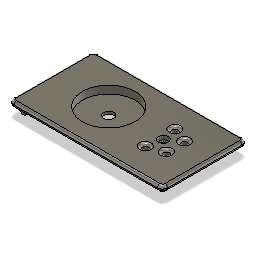
pluggable-12v-dimmer (Autodesk Fusion 360 design; units mm, degrees)
Autodesk Fusion 360 part; units mm, degrees
note: some values were not read from the file. Chosen so that the rebuilt part matches the saved one: which bodies a step acts on. Set by a fixed rule: which face or edge a step refers to.
sketch "pcb" plane through (0, 0, 0) normal (0, 1, 0) x (1, 0, 0) in component "Logic board"
  line L0 (0, 0) -> (53, 0)
  line L1 (53, 0) -> (53, -40)
  line L2 (53, -40) -> (0, -40)
  line L3 (0, -40) -> (0, 0)
  dimension "d1" = 53
  dimension "d2" = 40
  constraint horizontal L0
  constraint vertical L1
  constraint horizontal L2
  constraint vertical L3
  constraint coincident L0.start L3.end
  measures "d1" distance of L0.start L0.end
  measures "d2" distance of L0.start L2.end
sketch "esp32" plane through (0, 0, 0) normal (0, 1, 0) x (-1, 0, 0) in component "Logic board"
  line L0 (-3, -5) -> (-32, -5)
  line L1 (-32, -5) -> (-32, 47)
  line L2 (-32, 47) -> (-3, 47)
  line L3 (-3, 47) -> (-3, -5)
  dimension "d3" = 29
  dimension "d4" = 52
  constraint horizontal L0
  constraint vertical L1
  constraint horizontal L2
  constraint vertical L3
  measures "d3" distance of L0.start L0.end
  measures "d4" distance of L0.start L2.end
sketch "rotary enc" plane through (0, 0, 0) normal (0, 1, 0) x (1, 0, 0) in component "Logic board"
  circle A0 centre (40, -22) radius 6.5
  circle A1 centre (40, -22) radius 3.4
  point P0 (40, -22)
  dimension "d5" = 13
  dimension "d6" = 6.8
  constraint concentric A0 A1
  constraint coincident P0 A0.centre
  measures "d5" diameter of A0
  measures "d6" diameter of A1
sketch "Pololu" plane through (0, 0, 0) normal (0, 1, 0) x (1, 0, 0) in component "Logic board"
  line L0 (33, -15) -> (50, -15)
  line L1 (50, -15) -> (50, -2)
  line L2 (50, -2) -> (33, -2)
  line L3 (33, -2) -> (33, -15)
  dimension "d7" = 17
  constraint horizontal L0
  constraint vertical L1
  constraint horizontal L2
  constraint vertical L3
  measures "d7" distance of L0.start L0.end
sketch "mosfet" plane through (0, 0, 0) normal (0, 1, 0) x (1, 0, 0) in component "Logic board"
  line L0 (40, -30) -> (59, -30)
  line L1 (59, -30) -> (59, -39)
  line L2 (59, -39) -> (40, -39)
  line L3 (40, -39) -> (40, -30)
  constraint horizontal L0
  constraint vertical L1
  constraint horizontal L2
  constraint vertical L3
extrude "Extrude1" add sketch "pcb" against normal blind 2.5 makes body 1 in component "Logic board"
extrude "Extrude2" add sketch "esp32" along normal blind 7.5 bodies 1 in component "Logic board"
extrude "Extrude3" add sketch "rotary enc" sketch "mosfet" sketch "Pololu" along normal blind 6 contours A0 | A1 of sketch 2 of sketch 3 bodies 1 in component "Logic board"
extrude "Extrude4" add sketch "rotary enc" along normal blind 17.5 separate body contours A1 makes body 2 in component "Logic board"
sketch "jumper" plane through (0, 0, 0) normal (0, 1, 0) x (1, 0, 0) in component "Logic board"
  line L0 (50, -16) -> (52, -16)
  line L1 (52, -16) -> (52, -19)
  line L2 (52, -19) -> (50, -19)
  line L3 (50, -19) -> (50, -16)
  constraint horizontal L0
  constraint vertical L1
  constraint horizontal L2
  constraint vertical L3
extrude "Extrude5" add sketch "jumper" along normal blind 10 bodies 1 in component "Logic board"
combine "Combine1" operation add target body 1 tool bodies 2 in component "Logic board"
sketch "Sketch1" plane through (0, 0, 0) normal (0, 1, 0) x (1, 0, 0) in component "PTT stekker"
  line L0 (51.8, -11.4201) -> (51.8, -30.6799)
  line L1 (20.5424, -1.0921) -> (51.8, -11.4201)
  line L2 (20.5424, -41.0079) -> (51.8, -30.6799)
  arc A0 (20.5424, -1.0921) -> (20.5424, -41.0079) centre (21.0782, -21.05) ccw
  circle A1 centre (19.6032, -9.55) radius 2
  circle A2 centre (19.6032, -32.55) radius 2
  circle A3 centre (31.0676, -13.85) radius 2
  circle A4 centre (31.0676, -28.25) radius 2
  line L3 (21.0782, -40.35) -> (15.9681, -40.35)
  line L4 (21.0782, -40.35) -> (22.5334, -40.35)
  line L5 (21.0782, -1.75) -> (15.488, -1.8836)
  line L6 (21.0782, -1.75) -> (22.5334, -1.75)
  circle A5 centre (21.0782, -21.05) radius 4
  circle A6 centre (21.0782, -21.05) radius 2
  point P0 (19.6032, -9.55)
  point P1 (31.0676, -13.85)
  point P2 (31.0676, -28.25)
  point P3 (19.6032, -32.55)
  point P4 (21.0782, -21.05)
  dimension "d24" = 4
  dimension "d25" = 4
  dimension "d26" = 4
  dimension "d27" = 4
  dimension "d28" = 19.3
  dimension "d29" = 19.3
  dimension "d110" = 8
  dimension "d111" = 4
  constraint vertical L0
  constraint coincident P0 A1.centre
  constraint coincident P3 A2.centre
  constraint coincident P1 A3.centre
  constraint coincident P2 A4.centre
  constraint coincident A0 L3.end
  constraint coincident L2 L4.end
  constraint coincident A0 L5.end
  constraint coincident L1 L6.end
  constraint concentric A0 A5
  constraint concentric A0 A6
  constraint coincident P4 A0.centre
  measures "d24" diameter of A1
  measures "d25" diameter of A2
  measures "d26" diameter of A3
  measures "d27" diameter of A4
  measures "d28" distance of P4 L3.start
  measures "d29" distance of P4 L5.start
  measures "d110" diameter of A5
  measures "d111" diameter of A6
extrude "Extrude1'" add sketch "Sketch1" against normal blind 19.5 separate body contours A1 | A2 | A3 | A4 makes body 3 at (33.0651, -13, 28.3497) makes body 4 at (33.0651, -13, 13.9497) makes body 5 at (21.6007, -13, 32.6497) makes body 6 at (21.6007, -13, 9.6497) in component "PTT stekker"
extrude "Extrude2'" add sketch "Sketch1" along normal blind 12.5 contours L0 L1 L2 A0 L3 L4 L5 L6 | L1 A0 L5 L6 | L2 A0 L3 L4 | A1 | A2 | A3 | A4 | A5 | A6 bodies 3 4 5 6 in component "PTT stekker"
extrude "Extrude3'" cut sketch "Sketch1" along normal blind 9 contours L1 A0 L5 L6 | L2 A0 L3 L4 bodies 3 in component "PTT stekker"
extrude "Extrude4'" cut sketch "Sketch1" along normal blind 22 contours A6 bodies 3 in component "PTT stekker"
fillet "Fillet1" radius 2 4 edges at (29.2029, -19.5, 27.5268) (17.7386, -19.5, 31.8268) (17.7386, -19.5, 8.8268) (29.2029, -19.5, 13.1268) on bodies 3 4 5 6 in component "PTT stekker"
sketch "Sketch1 (2)" plane through (0, 0, 0) normal (0, 1, 0) x (1, 0, 0) in component "PTT stopcontact"
  line L0 (4, 0) -> (57.5, 0)
  line L1 (61.5, -4) -> (61.5, -57.5)
  line L2 (57.5, -61.5) -> (4, -61.5)
  line L3 (0, -57.5) -> (0, -4)
  arc A0 (4, 0) -> (0, -4) centre (4, -4) ccw
  arc A1 (61.5, -4) -> (57.5, 0) centre (57.5, -4) ccw
  arc A2 (57.5, -61.5) -> (61.5, -57.5) centre (57.5, -57.5) ccw
  arc A3 (0, -57.5) -> (4, -61.5) centre (4, -57.5) ccw
  circle A4 centre (29, -42.5) radius 3.5
  circle A5 centre (41, -38.4) radius 3.5
  circle A6 centre (41, -23.6) radius 3.5
  circle A7 centre (29, -19.5) radius 3.5
  circle A8 centre (29, -19.5) radius 2.2
  circle A9 centre (41, -23.6) radius 2.2
  circle A10 centre (29, -42.5) radius 2.2
  circle A11 centre (41, -38.4) radius 2.2
  line L4 (32.3924, -18.6389) -> (57.8397, -18.6389) construction
  circle A12 centre (31.4907, -30.8181) radius 3
  circle A13 centre (31.4907, -30.8181) radius 1.25
  arc A14 (59.75, -4) -> (57.5, -1.75) centre (57.5, -4) ccw
  line L5 (4, -1.75) -> (57.5, -1.75)
  arc A15 (4, -1.75) -> (1.75, -4) centre (4, -4) ccw
  line L6 (1.75, -57.5) -> (1.75, -4)
  arc A16 (1.75, -57.5) -> (4, -59.75) centre (4, -57.5) ccw
  line L7 (57.5, -59.75) -> (4, -59.75)
  arc A17 (57.5, -59.75) -> (59.75, -57.5) centre (57.5, -57.5) ccw
  line L8 (59.75, -4) -> (59.75, -57.5)
  line L9 (31.4907, -30.8181) -> (31.4907, -50.8681)
  line L10 (31.4907, -30.8181) -> (31.4907, -10.7681)
  circle A18 centre (31.4907, -50.8681) radius 2
  circle A19 centre (31.4907, -10.7681) radius 2
  point P0 (61.5, 0)
  point P1 (0, -61.5)
  point P2 (29, -19.5)
  point P3 (41, -23.6)
  point P4 (41, -38.4)
  point P5 (29, -42.5)
  dimension "d39" = 61.5
  dimension "d40" = 61.5
  dimension "d41" = 4
  dimension "d42" = 7
  dimension "d43" = 7
  dimension "d44" = 7
  dimension "d45" = 7
  dimension "d46" = 4.4
  dimension "d47" = 4.4
  dimension "d48" = 4.4
  dimension "d49" = 4.4
  dimension "d52" = 6
  dimension "d53" = 2.5
  dimension "d54" = 1.75
  dimension "d92" = 20.05
  dimension "d93" = 20.05
  dimension "d94" = 4
  dimension "d95" = 4
  constraint horizontal L0
  constraint vertical L1
  constraint horizontal L2
  constraint vertical L3
  constraint coincident origin L0
  constraint coincident origin L3
  constraint tangent L0 A0
  constraint tangent L3 A0
  constraint coincident P0 L0
  constraint coincident P0 L1
  constraint tangent L0 A1
  constraint tangent L1 A1
  constraint equal A0 A1
  constraint tangent L1 A2
  constraint tangent L2 A2
  constraint equal A0 A2
  constraint coincident P1 L2
  constraint coincident P1 L3
  constraint tangent L2 A3
  constraint tangent L3 A3
  constraint equal A0 A3
  constraint coincident P5 A4.centre
  constraint coincident P4 A5.centre
  constraint coincident P3 A6.centre
  constraint coincident P2 A7.centre
  constraint concentric A6 A9
  constraint concentric A4 A10
  constraint concentric A5 A11
  constraint horizontal L4
  constraint coincident A7 L4.start
  constraint concentric A12 A13
  constraint coincident A12.centre A13.centre
  constraint vertical L9
  constraint perpendicular L4 L10
  constraint coincident L9.end A18.centre
  constraint coincident L10.end A19.centre
  measures "d39" distance of origin P0
  measures "d40" distance of origin P1
  measures "d41" radius of A0
  measures "d42" diameter of A4
  measures "d43" diameter of A5
  measures "d44" diameter of A6
  measures "d45" diameter of A7
  measures "d46" diameter of A8
  measures "d47" diameter of A9
  measures "d48" diameter of A10
  measures "d49" diameter of A11
  measures "d52" diameter of A12
  measures "d53" diameter of A13
  measures "d92" distance of A12.centre L9.end
  measures "d93" distance of A12.centre L10.end
  measures "d94" diameter of A18
  measures "d95" diameter of A19
extrude "Extrude1''" add sketch "Sketch1 (2)" along normal blind 8.4 separate body contours L0 L1 L2 L3 A0 A1 A2 A3 | A4 L9 | A4 L9 | A5 | A6 | A7 L10 | A7 L10 | A8 | A9 | A10 | A11 | A12 A13 L9 L10 | A12 A13 L9 L10 | A13 L9 L10 | A13 L9 L10 | A14 L5 A15 L6 A16 L7 A17 L8 | A18 | A19 makes body 7 in component "PTT stopcontact"
extrude "Extrude2''" add sketch "Sketch1 (2)" along normal blind 9.1 contours A4 L9 | A4 L9 | A5 | A6 | A7 L10 | A7 L10 | A8 | A9 | A10 | A11 | A12 A13 L9 L10 | A12 A13 L9 L10 | A13 L9 L10 | A13 L9 L10 | A14 L5 A15 L6 A16 L7 A17 L8 | A18 | A19 bodies 7 in component "PTT stopcontact"
extrude "Extrude3''" add sketch "Sketch1 (2)" along normal blind 25.5 contours A4 L9 | A4 L9 | A5 | A6 | A7 L10 | A7 L10 | A12 A13 L9 L10 | A12 A13 L9 L10 bodies 7 in component "PTT stopcontact"
extrude "Extrude5'" cut sketch "Sketch1 (2)" along normal blind 10 contours A18 | A19 bodies 7 in component "PTT stopcontact"
move_body "Move1" bodies 7 to x (1, 0, 0) y (0, 1, 0) z (0, 0, 1) at (52, 0, -8) in component "PTT stopcontact"
move_body "Move1'" bodies 3 to x (1, 0, 0) y (0, 1, 0) z (0, 0, 1) at (0, 0, 2) in component "PTT stekker"
move_body "Move2" bodies 3 to x (1, 0, 0) y (0, 1, 0) z (0, 0, 1) at (0, -4, 0) in component "PTT stekker"
move_body "Move1''" bodies 1 to x (1, 0, 0) y (0, 1, 0) z (0, 0, 1) at (-1, 11, 0) in component "Logic board"
sketch "Sketch1 (3)" plane through (0, -4, 0) normal (0, -1, 0) x (1, 0, 0) in component "case"
  line L0 (22.5334, 42.35) -> (15.9681, 42.35)
  arc A0 (15.9681, 42.35) -> (15.488, 3.8836) centre (21.0782, 23.05) ccw
  line L1 (15.488, 3.8836) -> (21.0782, 3.75)
  line L2 (21.0782, 3.75) -> (22.5334, 3.75)
  line L3 (22.5334, 3.75) -> (51.8, 13.4201)
  line L4 (51.8, 13.4201) -> (51.8, 32.6799)
  line L5 (51.8, 32.6799) -> (22.5334, 42.35)
  circle A1 centre (19.6032, 11.55) radius 2
  circle A2 centre (19.6032, 34.55) radius 2
  circle A3 centre (31.0676, 15.85) radius 2
  circle A4 centre (31.0676, 30.25) radius 2
  line L6 (112, 56) -> (0, 56)
  line L7 (-4, 52) -> (-4, -6)
  line L8 (0, -10) -> (112, -10)
  line L9 (116, -6) -> (116, 52)
  arc A5 (0, 56) -> (-4, 52) centre (0, 52) ccw
  arc A6 (116, 52) -> (112, 56) centre (112, 52) ccw
  arc A7 (112, -10) -> (116, -6) centre (112, -6) ccw
  arc A8 (-4, -6) -> (0, -10) centre (0, -6) ccw
  line L10 (-1, 52) -> (-1, -6)
  arc A9 (-1, -6) -> (0, -7) centre (0, -6) ccw
  line L11 (0, -7) -> (112, -7)
  arc A10 (112, -7) -> (113, -6) centre (112, -6) ccw
  line L12 (113, -6) -> (113, 52)
  arc A11 (113, 52) -> (112, 53) centre (112, 52) ccw
  line L13 (112, 53) -> (0, 53)
  arc A12 (0, 53) -> (-1, 52) centre (0, 52) ccw
  line L14 (52, -8) -> (-2, -8)
  line L15 (-2, -8) -> (-2, 54)
  line L16 (-2, 54) -> (52, 54)
  line L17 (19.0543, 1.75) -> (22.8553, 1.75)
  line L18 (22.8553, 44.35) -> (15.7141, 44.35)
  arc A13 (15.7141, 44.35) -> (15.3765, 1.8379) centre (21.0782, 23.05) ccw
  line L19 (15.3765, 1.8379) -> (19.0543, 1.75)
  line L20 (22.8553, 1.75) -> (52, 11.3798)
  line L21 (52, 54) -> (52, 34.7202)
  line L22 (52, 11.3798) -> (52, -8)
  line L23 (52, 34.7202) -> (22.8553, 44.35)
  circle A14 centre (83.5, 2.7538) radius 1.9501
  circle A15 centre (83.5, 42.8333) radius 1.9003
  circle A16 centre (83.5, 2.7538) radius 1.4501
  circle A17 centre (83.5, 42.8333) radius 1.4003
  circle A18 centre (21.0782, 23.05) radius 2
  point P0 (116, 56)
  point P1 (-4, 56)
  point P2 (116, -10)
  dimension "d61" = 120
  dimension "d62" = 66
  dimension "d63" = 4
  dimension "d64" = 4
  dimension "d65" = 4
  dimension "d66" = 4
  dimension "d67" = -3
  dimension "d100" = -0.5
  dimension "d101" = -0.5
  constraint horizontal L6
  constraint vertical L7
  constraint horizontal L8
  constraint vertical L9
  constraint coincident P1 L6
  constraint coincident P1 L7
  constraint tangent L6 A5
  constraint tangent L7 A5
  constraint coincident P0 L6
  constraint coincident P0 L9
  constraint tangent L6 A6
  constraint tangent L9 A6
  constraint coincident P2 L9
  constraint coincident P2 L8
  constraint tangent L9 A7
  constraint tangent L8 A7
  constraint tangent L7 A8
  constraint tangent L8 A8
  constraint horizontal L14
  constraint vertical L15
  constraint horizontal L16
  constraint vertical L21
  constraint parallel L2 L17
  constraint parallel L0 L18
  constraint concentric A0 A13
  constraint parallel L1 L19
  constraint coincident L20.end L21
  constraint parallel L3 L20
  constraint parallel L5 L23
  measures "d61" distance of P0 P1
  measures "d62" distance of P0 P2
  measures "d63" radius of A5
  measures "d64" radius of A6
  measures "d65" radius of A7
  measures "d66" radius of A8
extrude "Extrude4''" add sketch "Sketch1 (3)" against normal blind 5 separate body contours A16 | A17 makes body 8 at (84.3174, -2.3333, 43.9703) makes body 9 at (82.4875, -0.6667, 3.7919) in component "case"
extrude "Extrude2'''" add sketch "Sketch1 (3)" against normal blind 15 separate body contours L10 A9 L11 L13 A12 L17 L18 A13 L19 L20 L21 L22 L23 makes body 10 in component "case"
extrude "Extrude1'''" add sketch "Sketch1 (3)" against normal blind 8.2 separate body contours L6 L7 L8 L9 A5 A6 A7 A8 | L10 A9 L11 L13 A12 L17 L18 A13 L19 L20 L21 L22 L23 | L10 A9 L11 L13 A12 L14 L15 L16 L21 L22 | L11 A10 L12 A11 L13 L17 L18 A13 L19 L20 L21 L22 L23 | A14 | A15 | A16 | A17 makes body 11 in component "case"
combine "Combine1'" operation cut target body 10 tool bodies 1 keep tools in component "case"
extrude "Extrude3'''" add sketch "Sketch1 (3)" against normal blind 37 contours L6 L7 L8 L9 A5 A6 A7 A8 | L10 A9 L11 L13 A12 L14 L15 L16 L21 L22 bodies 11 10 in component "case"
move_face "OffsetFaces1" offset -1 1 faces at (113, 13.8, 13.3333) on bodies 11 in component "case"
move_face "OffsetFaces2" offset -1 1 faces at (92.6667, 16.0667, -7) on bodies 11 in component "case"
move_face "OffsetFaces3" offset -1 1 faces at (92.6667, 16.0667, 53) on bodies 11 in component "case"
move_face "OffsetFaces4" offset -1 1 faces at (-1, 25.6667, 28.6667) on bodies 11 in component "case"
move_face "OffsetFaces5" offset -1 6 faces at (42.0445, -1.2667, 35.9033) (20.345, 1.4667, 42.35) (13.6718, 1.4667, 4.5096) (17.3514, -1.2667, 3.839) (21.5633, -1.2667, 3.75) (32.2889, -1.2667, 6.9734) on bodies 11 in component "case"
move_face "OffsetFaces6" offset 2 2 faces at (17.2455, -1.2667, 2.8413) (21.609, -1.2667, 2.75) on bodies 11 in component "case"
move_face "OffsetFaces7" offset 2 1 faces at (18.1245, 1.4667, 43.35) on bodies 11 in component "case"
chamfer "Chamfer1" distance 11 angle 20 1 edges at (52, 6.35, 11.3798) measured on face at (42.2851, 7.0667, 8.1699) on bodies 11 in component "case"
chamfer "Chamfer2" distance 3 angle 70 1 edges at (52, 6.35, 34.7202) measured on face at (52, 7.9, 49.3333) on bodies 11 in component "case"
move_face "OffsetFaces8" offset -1 2 faces at (17.5284, 1.4667, 4.8351) (26.1949, 1.4667, 4.75) on bodies 11 in component "case"
move_face "OffsetFaces9" offset -1 1 faces at (16.8149, 1.4667, 41.35) on bodies 11 in component "case"
move_face "OffsetFaces10" offset -0.5 1 faces at (51.8, -1.2667, 19.489) on bodies 11 in component "case"
move_face "OffsetFaces11" offset 7 4 faces at (16.3333, 11, -2.6667) (38.8035, 8.5, 3.2263) (44.0648, 8.5, 39.102) (24.6184, 11, 50.7833) on bodies 11 in component "case"
move_face "OffsetFaces12" offset -0.5 1 faces at (16, 17.1667, 0) on bodies 11 in component "case"
move_face "OffsetFaces13" offset -0.5 2 faces at (46.6735, 17.1667, 40) (4.0721, 17.1667, 40) on bodies 11 in component "case"
move_body "Move1'''" bodies 9 8 to x (1, 0, 0) y (0, 1, 0) z (0, 0, 1) at (0, 4, 0) in component "case"
combine "Combine2" operation cut target body 11 tool bodies 8 9 in component "case"
sketch "Sketch2" plane through (-2, 0, 0) normal (1, 0, 0) x (0, 0, -1) in component "case"
  line L0 (-53, 33) -> (-53, 18)
  line L1 (-53, 18) -> (-40.5, 18)
  line L2 (-40.5, 18) -> (-40.5, 15.5)
  line L3 (-40.5, 15.5) -> (0.5, 15.5)
  line L4 (0.5, 15.5) -> (0.5, 18)
  line L5 (0.5, 18) -> (7, 18)
  line L6 (7, 18) -> (7, 33)
  line L7 (7, 33) -> (-53, 33)
  line L8 (-40, 28) -> (-50, 28)
  line L9 (-50, 28) -> (-50, 25)
  line L10 (-50, 25) -> (-40, 25)
  line L11 (-40, 25) -> (-40, 28)
  line L12 (4, 28) -> (-6, 28)
  line L13 (-6, 28) -> (-6, 25)
  line L14 (-6, 25) -> (4, 25)
  line L15 (4, 25) -> (4, 28)
  constraint horizontal L8
  constraint vertical L9
  constraint horizontal L10
  constraint vertical L11
  constraint horizontal L12
  constraint vertical L13
  constraint horizontal L14
  constraint vertical L15
extrude "Extrude5''" cut sketch "Sketch2" against normal blind 1 contours L8 L9 L10 L11 | L12 L13 L14 L15 bodies 11 in component "case"
fillet "Fillet1'" radius 1 1 edges at (-3, 25, 1) on bodies 11 in component "case"
fillet "Fillet2" radius 1 1 edges at (-3, 25, 45) on bodies 11 in component "case"
fillet "Fillet3" radius 1 1 edges at (-3, 28, 1) on bodies 11 in component "case"
fillet "Fillet4" radius 1 1 edges at (-3, 28, 45) on bodies 11 in component "case"
sketch "Sketch1 (4)" plane through (0, 33, 0) normal (0, 1, 0) x (-1, 0, 0) in component "Lid"
  line L0 (1, -8) -> (-113, -8)
  arc A0 (-114, -7) -> (-113, -8) centre (-113, -7) ccw
  line L1 (-114, -7) -> (-114, 53)
  arc A1 (-113, 54) -> (-114, 53) centre (-113, 53) ccw
  line L2 (-113, 54) -> (1, 54)
  arc A2 (2, 53) -> (1, 54) centre (1, 53) ccw
  line L3 (2, 53) -> (2, -7)
  arc A3 (1, -8) -> (2, -7) centre (1, -7) ccw
  arc A4 (0, -10) -> (4, -6) centre (0, -6) ccw
  line L4 (4, -6) -> (4, 52)
  arc A5 (4, 52) -> (0, 56) centre (0, 52) ccw
  line L5 (0, 56) -> (-112, 56)
  arc A6 (-112, 56) -> (-116, 52) centre (-112, 52) ccw
  line L6 (-116, 52) -> (-116, -6)
  arc A7 (-116, -6) -> (-112, -10) centre (-112, -6) ccw
  line L7 (-112, -10) -> (0, -10)
  line L8 (1.5, -6) -> (1.5, 52)
  arc A8 (1.5, 52) -> (0, 53.5) centre (0, 52) ccw
  line L9 (0, 53.5) -> (-112, 53.5)
  arc A9 (-112, 53.5) -> (-113.5, 52) centre (-112, 52) ccw
  line L10 (-113.5, 52) -> (-113.5, -6)
  arc A10 (-113.5, -6) -> (-112, -7.5) centre (-112, -6) ccw
  line L11 (-112, -7.5) -> (0, -7.5)
  arc A11 (0, -7.5) -> (1.5, -6) centre (0, -6) ccw
  line L12 (1.5, -2.985) -> (-2, -2.985)
  line L13 (-2, -2.985) -> (-2, 5)
  line L14 (-2, 5) -> (1.5, 5)
  line L15 (1.5, 5) -> (1.5, -2.985)
  line L16 (1.5, 48.9374) -> (-2, 48.9374)
  line L17 (-2, 48.9374) -> (-2, 41)
  line L18 (-2, 41) -> (1.5, 41)
  line L19 (1.5, 41) -> (1.5, 48.9374)
  circle A12 centre (-40, 22) radius 20.5
  circle A13 centre (-40, 22) radius 4
  circle A14 centre (-40, 22) radius 22.5
  circle A15 centre (-81, 11.4165) radius 2.5
  circle A16 centre (-81, 34.4165) radius 2.5
  circle A17 centre (-93, 15.9165) radius 2.5
  circle A18 centre (-93, 30.1165) radius 2.5
  circle A19 centre (-83.5073, 22.86) radius 1.7867
  circle A20 centre (-83.5073, 22.86) radius 3.7867
  dimension "d114" = -2.5
  dimension "d136" = 41
  dimension "d137" = 8
  dimension "d138" = 2
  dimension "d156" = 5
  dimension "d157" = 5
  dimension "d158" = 5
  dimension "d159" = 5
  dimension "d160" = 3.5734
  dimension "d163" = 2
  constraint horizontal L12
  constraint vertical L13
  constraint horizontal L14
  constraint vertical L15
  constraint coincident L8 L12.start
  constraint horizontal L16
  constraint vertical L17
  constraint horizontal L18
  constraint vertical L19
  constraint coincident L8 L16.start
  constraint concentric A12 A13
  measures "d136" diameter of A12
  measures "d137" diameter of A13
  measures "d156" diameter of A15
  measures "d157" diameter of A16
  measures "d158" diameter of A17
  measures "d159" diameter of A18
  measures "d160" diameter of A19
extrude "Extrude8" add sketch "Sketch1 (4)" along normal blind 3 separate body contours A19 | A20 makes body 12 in component "Lid"
extrude "Extrude7" add sketch "Sketch1 (4)" along normal mid plane 8 separate body contours A15 | A16 | A17 | A18 | A19 makes body 13 at (83.0234, 35.6667, 24.5799) makes body 14 at (90.5124, 34.3333, 15.6676) makes body 15 at (78.5124, 34.3333, 34.1676) makes body 16 at (78.5124, 34.3333, 11.1676) makes body 17 at (90.5124, 34.3333, 29.8676) in component "Lid"
extrude "Extrude1''''" add sketch "Sketch1 (4)" along normal blind 3 separate body contours L0 A0 L1 A1 L2 A2 L3 A3 | A4 L4 A5 L5 A6 L6 A7 L7 | L8 A8 L9 A9 L10 A10 L11 A11 L12 L13 L14 L16 L17 L18 | L8 L12 L13 L14 L15 | L8 L16 L17 L18 L19 | A14 | A15 | A16 | A17 | A18 | A19 | A20 makes body 18 in component "Lid"
sketch "Sketch1 (5)" plane through (56, 33, 23) normal (0, 1, 0) x (-1, 0, 0) in component "Knob"
  circle A0 centre (16, -1) radius 3.05
  circle A1 centre (16, -1) radius 20
  circle A2 centre (16, -1) radius 18
  circle A3 centre (16, -1) radius 5.05
  line L0 (15.929, -4.0492) -> (15.929, 0.4508)
  line L1 (15.929, 0.4508) -> (18.6828, 0.4508)
  line L2 (15.929, 0.4508) -> (13.3172, 0.4508)
  point P0 (16, -1)
  dimension "d115" = 6.1
  dimension "d116" = 40
  dimension "d117" = -2
  dimension "d118" = 2
  dimension "d119" = 4.5
  dimension "d120" = 2.7539
  constraint concentric A0 A1
  constraint coincident A0 L0.start
  constraint vertical L0
  constraint coincident A0 L1.end
  constraint perpendicular L0 L1
  constraint coincident A0 L2.end
  constraint perpendicular L0 L2
  constraint coincident P0 A0.centre
  measures "d115" diameter of A0
  measures "d116" diameter of A1
  measures "d119" distance of L0.start L0.end
  measures "d120" distance of L0.end L1.end
extrude "Extrude1'''''" add sketch "Sketch1 (5)" along normal blind 3 separate body contours A0 L0 L1 | A0 L1 L2 | A0 L0 L2 | A1 | A2 | A3 makes body 19 in component "Knob"
extrude "Extrude2''''" add sketch "Sketch1 (5)" against normal blind 9 contours A1 bodies 19 in component "Knob"
extrude "Extrude3''''" add sketch "Sketch1 (5)" against normal blind 8 contours A0 L1 L2 | A3 bodies 19 in component "Knob"
fillet "Fillet1''" radius 1 1 edges at (58.6465, 36, 14.7677) on bodies 19 in component "Knob"
move_body "Move1''''" bodies 19 to x (1, 0, 0) y (0, 1, 0) z (0, 0, 1) at (0, 6, 0) in component "Knob"
sketch "Sketch3" plane through (0, 0, 42.35) normal (0, 0, -1) x (-1, 0, 0) in component "case"
  line L0 (-25.7208, -4) -> (-12.8902, -4)
  line L1 (-12.8902, -4) -> (-12.8902, 4.2)
  line L2 (-12.8902, 4.2) -> (-25.7208, 4.2)
  line L3 (-25.7208, 4.2) -> (-25.7208, -4)
  line L4 (-22.7075, 4.2) -> (-16, 4.2)
  line L5 (-16, 4.2) -> (-16, -4)
  line L6 (-16, -4) -> (-22.7075, -4)
  line L7 (-22.7075, -4) -> (-22.7075, 4.2)
  constraint horizontal L4
  constraint vertical L5
  constraint horizontal L6
  constraint vertical L7
  constraint coincident L2 L4.start
extrude "Extrude6" add sketch "Sketch3" along normal blind 0.5 contours L0 L2 L4 L5 L6 L7 bodies 11 in component "case"
fillet "Fillet5" radius 3 1 edges at (16, 0.1, 41.85) on bodies 11 in component "case"
fillet "Fillet6" radius 3 1 edges at (22.7075, 0.1, 41.85) on bodies 11 in component "case"
sketch "Sketch4" plane through (0.1016, 0, 4.2512) normal (0.023886, 0, 0.999715) x (0.999715, 0, -0.023886) in component "case"
  line L0 (12.3207, -4) -> (20.9826, -4)
  line L1 (20.9826, -4) -> (20.9826, 4.2)
  line L2 (20.9826, 4.2) -> (12.3207, 4.2)
  line L3 (12.3207, 4.2) -> (12.3207, -4)
  line L4 (15.0194, -4) -> (22.9626, -4)
  line L5 (22.9626, -4) -> (22.9626, 4.2)
  line L6 (22.9626, 4.2) -> (15.0194, 4.2)
  line L7 (15.0194, 4.2) -> (15.0194, -4)
  constraint horizontal L4
  constraint vertical L5
  constraint horizontal L6
  constraint vertical L7
  constraint coincident L0 L4.start
extrude "Extrude7'" add sketch "Sketch4" along normal blind 0.5 contours L0 L1 L2 L4 L6 L7 | L1 L4 L5 L6 bodies 11 in component "case"
fillet "Fillet7" radius 3 1 edges at (23.0695, 0.1, 4.2026) on bodies 11 in component "case"
fillet "Fillet8" radius 3 1 edges at (15.1287, 0.1, 4.3923) on bodies 11 in component "case"
extrude "Extrude2'''''" add sketch "Sketch1 (4)" against normal blind 2.5 contours L8 A8 L9 A9 L10 A10 L11 A11 L12 L13 L14 L16 L17 L18 | L8 L12 L13 L14 L15 | L8 L16 L17 L18 L19 | A14 | A15 | A16 | A17 | A18 | A19 | A20 bodies 18 in component "Lid"
extrude "Extrude3'''''" add sketch "Sketch1 (4)" against normal blind 9 contours L8 L12 L13 L14 L15 | L8 L16 L17 L18 L19 bodies 18 in component "Lid"
extrude "Extrude4'''" add sketch "Sketch1 (4)" against normal blind 5 contours A14 bodies 18 in component "Lid"
extrude "Extrude5'''" add sketch "Sketch1 (4)" against normal blind 2 separate body contours A12 | A14 makes body 20 in component "Lid"
move_body "Move1'''''" bodies 20 to x (1, 0, 0) y (0, 1, 0) z (0, 0, 1) at (0, -3, 0) in component "Lid"
combine "Combine1''" operation add target body 18 tool bodies 20 in component "Lid"
sketch "Sketch2 (2)" plane through (-1.5, 0, 0) normal (-1, 0, 0) x (0, 0, 1) in component "Lid"
  line L0 (52, 33) -> (-6, 33)
  line L1 (-6, 33) -> (-6, 30.5)
  line L2 (-6, 30.5) -> (-2.985, 30.5)
  line L3 (-2.985, 30.5) -> (-2.985, 24)
  line L4 (-2.985, 24) -> (5, 24)
  line L5 (5, 24) -> (5, 30.5)
  line L6 (5, 30.5) -> (41, 30.5)
  line L7 (41, 30.5) -> (41, 24)
  line L8 (41, 24) -> (48.9374, 24)
  line L9 (48.9374, 24) -> (48.9374, 30.5)
  line L10 (48.9374, 30.5) -> (52, 30.5)
  line L11 (52, 30.5) -> (52, 33)
  line L12 (-3, 28) -> (5, 28)
  line L13 (5, 28) -> (5, 25)
  line L14 (5, 25) -> (-3, 25)
  line L15 (-3, 25) -> (-3, 28)
  line L16 (41, 28) -> (48.9374, 28)
  line L17 (48.9374, 28) -> (48.9374, 25)
  line L18 (48.9374, 25) -> (41, 25)
  line L19 (41, 25) -> (41, 28)
  constraint horizontal L12
  constraint vertical L13
  constraint horizontal L14
  constraint vertical L15
  constraint coincident L5 L13.end
  constraint horizontal L16
  constraint vertical L17
  constraint horizontal L18
  constraint vertical L19
  constraint coincident L9 L17.end
  constraint coincident L7 L16.start
extrude "Extrude6'" add sketch "Sketch2 (2)" along normal blind 1.2 contours L7 L9 L16 L17 L18 L19 | L3 L5 L12 L13 L14 bodies 18 in component "Lid"
fillet "Fillet1'''" radius 1.5 4 edges at (-2.7, 25, 1.0075) (-2.7, 25, 44.9687) (-2.7, 28, 44.9687) (-2.7, 28, 1.0075) on bodies 18 in component "Lid"
fillet "Fillet2'" radius 1 2 edges at (2, 24, 1.0075) (2, 24, 44.9687) on bodies 18 in component "Lid"
fillet "Fillet3'" radius 1 2 edges at (2, 30.5, 44.9687) (2, 30.5, 1.0075) on bodies 18 in component "Lid"
fillet "Fillet4'" radius 1 4 edges at (0.75, 30.5, -2.985) (0.75, 30.5, 41) (0.75, 30.5, 5) (0.75, 30.5, 48.9374) on bodies 18 in component "Lid"
fillet "Fillet5'" radius 2 8 edges at (116, 36, 23) (114.8284, 36, -8.8284) (56, 36, -10) (-2.8284, 36, -8.8284) (-4, 36, 23) (-2.8284, 36, 54.8284) (56, 36, 56) (114.8284, 36, 54.8284) on bodies 18 in component "Lid"
combine "Combine2'" operation cut target body 18 tool bodies 13 14 15 16 17 in component "Lid"
combine "Combine3" operation cut target body 18 tool bodies 12 in component "Lid"
fillet "Fillet6'" radius 2 4 edges at (83.3308, 36, 12.3206) (95.3308, 36, 16.8206) (95.3308, 36, 31.0206) (83.3308, 36, 35.3206) on bodies 18 in component "Lid"
component "Logic board" placed x (1, 0, 0) y (0, 1, 0) z (0, 0, 1) at (0, 0, 0)
component "PTT stekker" placed x (1, 0, 0) y (0, 1, 0) z (0, 0, 1) at (0, 0, 0)
component "case" placed x (1, 0, 0) y (0, 1, 0) z (0, 0, 1) at (0, 0, 0)
component "Lid" placed x (1, 0, 0) y (0, 1, 0) z (0, 0, 1) at (0, 0, 0)
component "Knob" placed x (1, 0, 0) y (0, 1, 0) z (0, 0, 1) at (0, 0, 0)
component "PTT stopcontact" placed x (1, 0, 0) y (0, 1, 0) z (0, 0, 1) at (0, 0, 0)
named bodies: "Logic board", "PTT Stekker", "PTT stopcontact"
